Autodesk Fusion 360 part; units mm, degrees
(part 2 of 2)
  constraint tangent L108 A249
  constraint tangent L109 A249
  constraint perpendicular L217 L244
  constraint perpendicular L234 L245
  constraint collinear L246 L247
  constraint collinear L248 L249
  constraint tangent L244 A250
  constraint tangent L247 A250
  constraint tangent L244 A251
  constraint tangent L248 A251
  constraint tangent L245 A252
  constraint tangent L246 A252
  constraint tangent L245 A253
  constraint tangent L249 A253
  constraint tangent A240 L251
  constraint tangent L237 A254
  constraint tangent L256 A254
  constraint tangent L236 A255
  constraint tangent L255 A255
  constraint tangent L236 A256
  constraint tangent L256 A256
  constraint tangent L235 A257
  constraint tangent L255 A257
  constraint tangent L233 A258
  constraint tangent L254 A258
  constraint tangent L232 A259
  constraint tangent L254 A259
  constraint tangent L231 A260
  constraint tangent L252 A260
  constraint tangent L231 A261
  constraint tangent L253 A261
  constraint tangent L232 A262
  constraint tangent L253 A262
  constraint tangent L230 A263
  constraint tangent L252 A263
  constraint tangent L230 A264
  constraint tangent L251 A264
  constraint tangent L229 A265
  constraint tangent L250 A265
  constraint tangent L241 A266
  constraint tangent L250 A266
  measures "d1" diameter of A0
  measures "d2" diameter of A1
  measures "d3" diameter of A2
  measures "d4" diameter of A3
  measures "d5" diameter of A4
  measures "d9" diameter of A111
  measures "d12" diameter of A112
extrude "Extrude1" add sketch "mriya" along normal blind 10.6 contours L106 L107 L216 A223 L217 L233 L234 A239 | L106 L107 L207 A214 L208 A215 L209 A216 L210 A217 L211 A218 L212 A219 L213 A220 L214 A221 L215 A222 L216 L217 A224 L218 A225 L219 A226 L220 A227 L221 A228 L222 A229 L223 A230 L224 A231 L225 A232 L226 A233 L227 A234 L228 A235 L229 L230 L231 L232 L233 L234 L235 L236 L237 L238 L239 L240 L241 L242 L243 A236 A237 A238 A240 A241 A242 A243 A244 L250 L251 L252 L253 L254 L255 L256 A254 A255 A256 A257 A258 A259 A260 A261 A262 A263 A264 A265 A266 makes body 1
extrude "Extrude2" add sketch "mriya" along normal blind 17.1 contours L106 L107 L216 A223 L217 L233 L234 A239 bodies 1
extrude "Extrude3" add sketch "mriya" along normal blind 2 from surface at 1.7 contours L108 L109 L110 L207 A214 L208 A215 L209 A216 L210 A217 L211 A218 L212 A219 L213 A220 L214 A221 L215 A222 L216 L217 A224 L218 A225 L219 A226 L220 A227 L221 A228 L222 A229 L223 A230 L224 A231 L225 A232 L226 A233 L227 A234 L228 A235 A245 A246 A247 A248 A249 | L110 L217 A247 A248 | L108 L109 L216 A223 L217 A245 A246 A249 | A114 | A115 | A116 | A117 bodies 1
extrude "Extrude6" add sketch "mriya" along normal blind 1 from surface at 14.3 contours L108 L109 L216 A223 L217 A245 A246 A249 bodies 1
extrude "Extrude7" add sketch "mriya" along normal blind 1 from surface at 7.8 contours L110 L217 A247 A248 bodies 1
chamfer "Chamfer5" distance 0.75 angle 45 4 edges at (-7, 57.2432, 14.3) (-7.4686, 77.6246, 14.3) (-15.85, 78.0932, 14.3) (-7, 9.5932, 7.8) on bodies 1
sketch "power-switch" plane through (-4.5, 0, 0) normal (1, 0, 0) x (0, 1, 0)
  line L0 (1.9932, 0) -> (76.4932, 0)
  line L1 (76.4932, 0) -> (76.4932, 17)
  line L2 (76.4932, 17) -> (19.2932, 17)
  line L3 (19.2932, 17) -> (19.2932, 10.5)
  line L4 (19.2932, 10.5) -> (1.9932, 10.5)
  line L5 (1.9932, 10.5) -> (1.9932, 0)
  line L6 (35.9932, 5.2) -> (25.7932, 5.2)
  line L7 (25.7932, 5.2) -> (25.7932, 7.9)
  line L8 (25.7932, 7.9) -> (35.9932, 7.9)
  line L9 (35.9932, 7.9) -> (35.9932, 5.2)
  line L10 (37.3932, 2.8) -> (24.3932, 2.8)
  line L11 (23.3932, 3.8) -> (23.3932, 9.3)
  line L12 (24.3932, 10.3) -> (37.3932, 10.3)
  line L13 (38.3932, 9.3) -> (38.3932, 3.8)
  arc A0 (24.3932, 10.3) -> (23.3932, 9.3) centre (24.3932, 9.3) ccw
  arc A1 (38.3932, 9.3) -> (37.3932, 10.3) centre (37.3932, 9.3) ccw
  arc A2 (37.3932, 2.8) -> (38.3932, 3.8) centre (37.3932, 3.8) ccw
  arc A3 (23.3932, 3.8) -> (24.3932, 2.8) centre (24.3932, 3.8) ccw
  line L14 (19.2932, 10.6) -> (1.8932, 10.6)
  line L15 (1.8932, 10.6) -> (1.8932, 0)
  line L16 (1.8932, 0) -> (76.5932, 0)
  line L17 (76.5932, 0) -> (76.5932, 17.1)
  line L18 (76.5932, 17.1) -> (19.2932, 17.1)
  line L19 (19.2932, 17.1) -> (19.2932, 10.6)
  constraint perpendicular L6 L7
  constraint tangent L11 A0
  constraint tangent L12 A0
  constraint tangent L12 A1
  constraint tangent L13 A1
  constraint tangent L10 A2
  constraint tangent L13 A2
  constraint tangent L10 A3
  constraint tangent L11 A3
  constraint vertical L7
  constraint perpendicular L7 L8
  constraint vertical L9
extrude "Extrude8" cut sketch "power-switch" against normal blind 2.5 contours L6 L7 L8 L9 bodies 1
extrude "Extrude9" cut sketch "power-switch" against normal blind 1 contours L10 L11 L12 L13 A0 A1 A2 A3 bodies 1
fillet "Fillet23" radius 0.1 8 edges at (-4.5, 23.3932, 6.55) (-4.5, 23.6861, 10.0071) (-4.5, 30.8932, 10.3) (-4.5, 38.1003, 10.0071) (-4.5, 38.3932, 6.55) (-4.5, 38.1003, 3.0929) (-4.5, 30.8932, 2.8) (-4.5, 23.6861, 3.0929) on bodies 1
fillet "Fillet24" radius 1 8 edges at (-5.5, 30.8932, 2.8) (-5.5, 23.6861, 3.0929) (-5.5, 23.3932, 6.55) (-5.5, 23.6861, 10.0071) (-5.5, 30.8932, 10.3) (-5.5, 38.1003, 10.0071) (-5.5, 38.3932, 6.55) (-5.5, 38.1003, 3.0929) on bodies 1
chamfer "Chamfer4" distance 0.8 angle 45 4 edges at (-7, 30.8932, 5.2) (-7, 35.9932, 6.55) (-7, 30.8932, 7.9) (-7, 25.7932, 6.55) on bodies 1
sketch "usb-c" plane through (0, 80.5932, 0) normal (0, 1, 0) x (-1, 0, 0)
  line L0 (3.6, 0) -> (36.1295, 0)
  line L1 (3.6, 16.7) -> (3.6, 0)
  line L2 (21.2002, 10.9) -> (21.2002, 10.1)
  arc A0 (21.2002, 10.9) -> (19.8003, 12.3) centre (19.8003, 10.9) ccw
  line L3 (11.8003, 10.1) -> (11.8003, 10.9)
  line L4 (19.8003, 8.7) -> (13.2003, 8.7)
  line L5 (19.7003, 7) -> (13.3002, 7)
  arc A1 (11.8003, 10.1) -> (13.2003, 8.7) centre (13.2003, 10.1) ccw
  line L6 (22.7003, 11) -> (22.7003, 10)
  line L7 (13.3002, 14) -> (19.7003, 14)
  arc A2 (13.2002, 12.3) -> (11.8002, 10.9) centre (13.2002, 10.9) ccw
  arc A3 (19.8003, 8.7) -> (21.2003, 10.1) centre (19.8003, 10.1) ccw
  line L8 (10.3002, 10) -> (10.3002, 11)
  line L9 (13.2002, 12.3) -> (19.8003, 12.3)
  line L10 (8.6, 0) -> (41.1295, 0)
  line L11 (41.1295, 10.5) -> (25.8, 10.5)
  line L12 (25.8, 10.5) -> (25.8, 17)
  line L13 (25.8, 17) -> (8.6, 17)
  line L14 (8.6, 17) -> (8.6, 0)
  line L15 (41.1295, 0) -> (41.1295, 10.5)
  arc A4 (13.3002, 14) -> (10.3002, 11) centre (13.3002, 11) ccw
  arc A5 (22.7003, 11) -> (19.7003, 14) centre (19.7003, 11) ccw
  arc A6 (10.3002, 10) -> (13.3002, 7) centre (13.3003, 10) ccw
  arc A7 (19.7003, 7) -> (22.7003, 10) centre (19.7003, 10) ccw
  line L16 (8.5, 0) -> (40.9017, 0)
  line L17 (40.9017, 10.6) -> (25.8, 10.6)
  line L18 (25.8, 10.6) -> (25.8, 17.1)
  line L19 (25.8, 17.1) -> (8.5, 17.1)
  line L20 (8.5, 17.1) -> (8.5, 0)
  line L21 (40.9017, 0) -> (40.9017, 10.6)
  constraint tangent L3 A2
  constraint tangent A2 L9
  constraint tangent A0 L9
  constraint tangent L2 A0
  constraint tangent L4 A3
  constraint tangent L2 A3
  constraint tangent L4 A1
  constraint tangent L3 A1
  constraint perpendicular L6 L7
  constraint perpendicular L5 L8
  constraint horizontal L5
  constraint perpendicular L5 L6
  constraint tangent L8 A4
  constraint tangent L7 A4
  constraint tangent L7 A5
  constraint tangent L6 A5
  constraint tangent L5 A6
  constraint tangent L8 A6
  constraint tangent L6 A7
  constraint tangent L5 A7
extrude "Extrude10" cut sketch "usb-c" against normal blind 2.5 contours L2 A0 L3 L4 A1 A2 A3 L9 bodies 1
extrude "Extrude11" cut sketch "usb-c" against normal blind 1.2 contours L5 L6 L7 L8 A4 A5 A6 A7 bodies 1
fillet "Fillet16" radius 0.1 8 edges at (-11.1789, 80.5932, 7.8787) (-10.3003, 80.5932, 10.5) (-11.1789, 80.5932, 13.1213) (-16.5003, 80.5932, 14) (-21.8216, 80.5932, 13.1213) (-22.7003, 80.5932, 10.5) (-21.8216, 80.5932, 7.8787) (-16.5003, 80.5932, 7) on bodies 1
fillet "Fillet20" radius 1.2 8 edges at (-16.5003, 79.3932, 7) (-11.1789, 79.3932, 7.8787) (-10.3003, 79.3932, 10.5) (-11.1789, 79.3932, 13.1213) (-16.5003, 79.3932, 14) (-21.8216, 79.3932, 13.1213) (-22.7003, 79.3932, 10.5) (-21.8216, 79.3932, 7.8787) on bodies 1
fillet "Fillet27" radius 1.5 90 edges at (-4.5, 47.9432, 17.1) (-5.6716, 79.4216, 17.1) (-17.15, 80.5932, 17.1) (-33.3509, 80.5932, 10.6) (-41.4757, 80.7074, 10.6) (-42.3069, 81.3771, 10.6) (-43.9492, 82.5887, 10.6) (-51.5908, 82.8932, 10.6) (-58.2758, 83.0074, 10.6) (-60.2069, 84.7771, 10.6) (-62.9492, 87.0887, 10.6) (-73.4, 87.3932, 10.6) (-83.8508, 87.0887, 10.6) (-86.0931, 85.2771, 10.6) (-87.5243, 84.0074, 10.6) (-94.7092, 83.8932, 10.6) (-102.8508, 83.5887, 10.6) (-107.3431, 79.5271, 10.6) (-111.0243, 76.0074, 10.6) (-115.9592, 75.8932, 10.6) (-121.8508, 75.5887, 10.6) (-123.4931, 74.3771, 10.6) (-124.3243, 73.7074, 10.6) (-131.5491, 73.5932, 10.6) (-141.0284, 72.4216, 10.6) (-142.2, 42.8932, 10.6) (-141.0284, 13.3648, 10.6) (-120.4435, 12.1932, 10.6) (-100.9649, 12.5357, 10.6) (-96.4569, 16.5593, 10.6) (-92.76, 20.041, 10.6) (-84.5813, 20.1932, 10.6) (-75.6559, 19.7842, 10.6) (-70.5608, 11.5973, 10.6) (-65.0991, 3.0385, 10.6) (-55.9906, 2.4932, 10.6) (-48.3243, 2.379, 10.6) (-47.4931, 1.7093, 10.6) (-45.8508, 0.4977, 10.6) (-37.1092, 0.1932, 10.6) (-29.3243, 0.079, 10.6) (-28.4931, -0.5907, 10.6) (-26.8508, -1.8023, 10.6) (-16.91, -2.1068, 10.6) (-5.6716, -0.9352, 10.6) (-4.5, 10.5932, 10.6) (-24.7009, 80.5932, 0) (-5.6716, 79.4216, 0) (-4.5, 39.2432, 0) (-5.6716, -0.9352, 0) (-16.91, -2.1068, 0) (-26.8508, -1.8023, 0) (-28.4931, -0.5907, 0) (-29.3243, 0.079, 0) (-37.1092, 0.1932, 0) (-45.8508, 0.4977, 0) (-47.4931, 1.7093, 0) (-48.3243, 2.379, 0) (-55.9906, 2.4932, 0) (-65.0991, 3.0385, 0) (-70.5608, 11.5973, 0) (-75.6559, 19.7842, 0) (-84.5813, 20.1932, 0) (-92.76, 20.041, 0) (-96.4569, 16.5593, 0) (-100.9649, 12.5357, 0) (-120.4435, 12.1932, 0) (-141.0284, 13.3648, 0) (-142.2, 42.8932, 0) (-141.0284, 72.4216, 0) (-131.5491, 73.5932, 0) (-124.3243, 73.7074, 0) (-123.4931, 74.3771, 0) (-121.8508, 75.5887, 0) (-115.9592, 75.8932, 0) (-111.0243, 76.0074, 0) (-107.3431, 79.5271, 0) (-102.8508, 83.5887, 0) (-94.7092, 83.8932, 0) (-87.5243, 84.0074, 0) (-86.0931, 85.2771, 0) (-83.8508, 87.0887, 0) (-73.4, 87.3932, 0) (-62.9492, 87.0887, 0) (-60.2069, 84.7771, 0) (-58.2758, 83.0074, 0) (-51.5908, 82.8932, 0) (-43.9492, 82.5887, 0) (-42.3069, 81.3771, 0) (-41.4757, 80.7074, 0) on bodies 1
chamfer "Chamfer6" distance 0.5 angle 45 6 edges at (-4.5, 19.2932, 12.35) (-4.9393, 19.2932, 16.6607) (-6.5, 19.2932, 17.1) (-25.8, 80.5932, 12.35) (-25.8, 80.1539, 16.6607) (-25.8, 78.5932, 17.1) on bodies 1
mirror "Mirror1" about plane through (0, 0, 0) normal (1, 0, 0) of bodies 1 makes body 2
named bodies: "Left", "Right"
